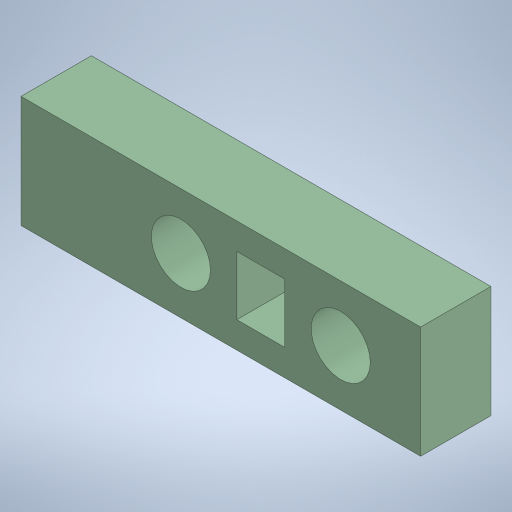
# Autodesk Inventor part: griper_base_TPU
Saved by Autodesk Inventor 2024 (Build 280153000, 153)
## iProperties
Created: 2025-06-02
Part Number: griper_base_TPU
Material: ゴム、シリコーン
Document SubType Name: Modeling
Designer: 1412z
Density: 1.25 g/cm^3
Appearance: ゴム - 緑
Author: 1412z
Autodesk Inventor part; units mm, degrees
ref_plane "YZ Plane" through (0, 0, 0) normal (1, 0, 0) x (0, 1, 0)
ref_plane "XZ Plane" through (0, 0, 0) normal (0, 1, 0) x (-1, 0, 0)
ref_plane "XY Plane" through (0, 0, 0) normal (0, 0, 1) x (1, 0, 0)
sketch "スケッチ1" plane through (0, 0, 0) normal (0, 0, 1) x (1, 0, 0)
  line L0 (12.5, -3.5) -> (-12.5, -3.5)
  line L1 (-12.5, -3.5) -> (-12.5, 3.5)
  line L2 (-12.5, 3.5) -> (12.5, 3.5)
  line L3 (12.5, 3.5) -> (12.5, -3.5)
  line L4 (12.5, -3.5) -> (-12.5, 3.5) construction
  line L5 (-12.5, -3.5) -> (12.5, 3.5) construction
  circle A0 centre (7.5, 0) radius 1.85
  circle A1 centre (-2.5, 0) radius 1.85
  line L6 (-2.5, 0) -> (7.5, 0)
  line L7 (2.5, 1.85) -> (4, 1.85)
  line L8 (4, 1.85) -> (4, -1.85)
  line L9 (4, -1.85) -> (1, -1.85)
  line L10 (1, -1.85) -> (1, 1.85)
  line L11 (1, 1.85) -> (2.5, 1.85)
  point P0 (0, 0)
  dimension "d0" = 25
  dimension "d1" = 7
  dimension "d2" = 3.7
  dimension "d3" = 3.7
  dimension "d6" = 1.5
  dimension "d7" = 3
  constraints: 24 end point, 5 perpendicular, 3 parallel, 2 centre point, 2 horizontal, 2 midpoint, 1 point on line
  measures "d0" distance of L1.end L2.end
  measures "d1" distance of L0.end L1.end
  measures "d2" diameter of A0
  measures "d3" diameter of A1
  measures "d6" distance of L7.start L7.end
  measures "d7" distance of L8.end L9.end
extrude "押し出し1" add sketch "スケッチ1" along normal blind 4.4 contours L0 L1 L2 L3 | L8 L9 L10 L6 | L6 L10 L11 L7 L8
sketch "スケッチ2" plane through (0, 0, 4.4) normal (0, 0, 1) x (1, 0, 0)
  line L0 (2.5, 1.85) -> (4, 1.85)
  line L1 (4, 1.85) -> (4, -1.85)
  line L2 (4, -1.85) -> (1, -1.85)
  line L3 (1, -1.85) -> (1, 1.85)
  line L4 (1, 1.85) -> (2.5, 1.85)
  point P0 (0, 0)
  dimension "d8" = 1.5
  dimension "d9" = 3
  constraints: 10 end point, 4 perpendicular, 1 horizontal, 1 point on line
  measures "d8" distance of L0.start L0.end
  measures "d9" distance of L1.end L2.end
extrude "押し出し2" cut sketch "スケッチ2" against normal blind 10
